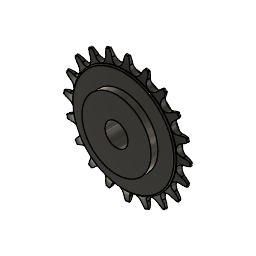
2410994757_Bicycle-sprocket1 (Autodesk Fusion 360 design; units mm, degrees)
part number: 2025-11-01-18-05-41-506
Autodesk Fusion 360 part; units mm, degrees
sketch "Sketch1" plane through (0, 0, 0) normal (0, 1, 0) x (1, 0, 0)
  circle A0 centre (0, 0) radius 37.5
  circle A1 centre (0, 0) radius 33.75
  circle A2 centre (0, 0) radius 41.6667
  line L0 (0, 0) -> (0, -48.246)
  line L1 (0, 0) -> (-7.6961, -48.5915)
  circle A3 centre (-5.8663, -37.0383) radius 3.75
  circle A4 centre (5.8663, -37.0383) radius 3.75
  circle A5 centre (9.5362, -36.2672) radius 11.6717
  circle A6 centre (-9.5362, -36.2672) radius 11.6717
  arc A7 (-1.0259, -41.2344) -> (-0.3536, -41.6652) centre (-0.3472, -40.9152) ccw
  arc A8 (0.3536, -41.6652) -> (1.0259, -41.2344) centre (0.3472, -40.9152) ccw
  dimension "d1" = 75
  dimension "d3" = 67.5
  dimension "d4" = 83.3333
  dimension "d5" = 9
  dimension "d6" = 1.5
  constraint coincident A0.centre A1.centre
  constraint concentric A0 A1
  constraint concentric A1 A2
  constraint vertical L0
  constraint coincident A0 A3.centre
  constraint coincident L1 A3.centre
  constraint tangent A1 A3
  constraint symmetric L0 A3 A4
  constraint coincident A4 A5.centre
  constraint coincident A0 A5.centre
  constraint tangent A3 A5
  constraint symmetric L0 A5 A6
  constraint tangent A5 A7
  constraint tangent A2 A7
  constraint symmetric L0 A7 A8
  constraint coincident A5 A7.start
  constraint coincident A6 A8.end
  constraint coincident A2 A7.end
  constraint coincident A2 A8.start
  measures "d1" diameter of A0
  measures "d3" diameter of A1
  measures "d4" diameter of A2
  measures "d5" angle of L0 L1
  measures "d6" diameter of A7
extrude "Extrude1" add sketch "Sketch1" along normal mid plane 6 contours A1 A3 A5 | A1 A4 A6 | A0 A1 L0 A5 | A0 A2 L0 A6 A8 | A0 A1 L0 A6 | A0 A2 L0 A5 A7 makes body 1
extrude "Extrude2" add sketch "Sketch1" along normal mid plane 6 separate body contours A1 L1 A6 | A1 L0 L1 A5 A6 | A1 A5 A6 | A1 L1 A5 A6 | L0 L1 A6 | A1 L0 A6 | A1 L0 A5 makes body 2
sketch "Sketch2" plane through (0, 0, 0) normal (1, 0, 0) x (0, 1, 0)
  line L0 (0, 0) -> (0, 50)
  line L1 (3, 0) -> (3, 60)
  line L2 (-3, 0) -> (-3, 60)
  arc A0 (-2.0965, 33.3228) -> (-0.6531, 41.0213) centre (-23.3532, 41.2928) ccw
  arc A1 (0.6531, 41.0213) -> (2.0965, 33.3228) centre (23.3532, 41.2928) ccw
  circle A2 centre (0, 0) radius 33.75
  line L3 (-9, 52) -> (-8, 52)
  line L4 (-8, 52) -> (27, 52)
  arc A3 (-3, 41.5585) -> (3, 41.5585) centre (0, 0) ccw
  arc A4 (0, 41.6667) -> (-0.6545, 41.6615) centre (0, 0) ccw
  line L5 (0, 0) -> (-0.5301, 33.7458)
  line L6 (-0.6543, 41.6494) -> (-0.7647, 48.6769)
  arc A5 (0.6531, 41.0213) -> (-0.6531, 41.0213) centre (0, 41.0135) ccw
  line L7 (-50, 0) -> (55, 0)
  dimension "d11" = 0.9
  dimension "d13" = 83.3333
  dimension "d14" = 67.5
  constraint coincident L0.start A2.centre
  constraint vertical L0
  constraint symmetric L0 L1.start L2.start
  constraint symmetric L0 L1.end L2.end
  constraint tangent A0 L5
  constraint coincident L6.start L5
  constraint symmetric L0 A0.start A1.end
  constraint symmetric L0 A0 A1
  constraint horizontal L3
  constraint parallel L3 L4
  constraint coincident L0 A5.centre
  constraint tangent A0 A5
  constraint tangent A3 A5
  constraint coincident A4.end L5
  constraint coincident L2 A3.start
  constraint coincident L1 A3.end
  constraint coincident L0 A4.start
  constraint concentric A3 A4
  constraint collinear L5 L6
  constraint coincident A2 L5.end
  constraint horizontal L7
  measures "d11" angle of L0 L5
  measures "d13" diameter of A3
  measures "d14" diameter of A2
revolve "Revolve1" cut sketch "Sketch2" angle 360 about axis through (0, -50, 0) along (0, 1, 0) contours L1 L2 A0 A1 A2 L4 A5 | L2 A2 A3 L7 | L1 A2 A3 L7 bodies 1 2
fillet "Fillet1" radius 0.75 2 edges at (12.1562, -3, -31.3415) (12.1562, 3, 31.3415) on bodies 2
sketch "Sketch3" plane through (0, 0, 0) normal (0, 1, 0) x (1, 0, 0)
  circle A0 centre (0, 0) radius 7.5
  circle A1 centre (0, 0) radius 22.5
  dimension "d18" = 15
  dimension "d19" = 45
  constraint coincident A0.centre A1.centre
  measures "d18" diameter of A0
  measures "d19" diameter of A1
extrude "Extrude3" add sketch "Sketch3" along normal mid plane 15 separate body makes body 3
extrude "Extrude4" cut sketch "Sketch3" along normal mid plane 40 contours A0 bodies 2
pattern_circular "C-Pattern1" count 20 over 360 about axis through (0, -3, 0) along (0, 1, 0) of bodies 1 makes body 4 at (6.4398, 0.6471, 33.1299) makes body 5 at (17.3825, -0.6471, 28.9294) makes body 6 at (28.9294, 0.6471, 17.3825) makes body 7 at (31.067, -0.6471, 13.1872) makes body 8 at (33.6216, -0.6471, 2.9415) makes body 9 at (33.1299, 0.6471, -6.4398) makes body 10 at (29.5184, 0.6471, -16.3623) makes body 11 at (22.142, -0.6471, -25.4714) makes body 12 at (13.1872, -0.6471, -31.067) makes body 13 at (2.9415, -0.6471, -33.6216) makes body 14 at (-7.5921, -0.6471, -32.885) makes body 15 at (-16.3623, 0.6471, -29.5184) makes body 16 at (-25.4714, -0.6471, -22.142) makes body 17 at (-31.067, -0.6471, -13.1872) makes body 18 at (-33.6216, -0.6471, -2.9415) makes body 19 at (-32.885, -0.6471, 7.5921) makes body 20 at (-28.9294, -0.6471, 17.3825) makes body 21 at (-22.142, -0.6471, 25.4714) makes body 22 at (-13.1872, -0.6471, 31.067)
combine "Combine1" operation add target body 12 tool bodies 4 8 11 18 14 2 15 1 19 3 5 22 20 13 16 9 17 10 7 21 6
equation "d3 = ( 75 * 0.9 ) * 1 mm"
equation "d4 = ( 75 / 0.9 ) * 1 mm"
equation "d7 = 2 * 1.5 mm"
equation "d9 = 2 * 1.5 mm"
equation "d13 = ( 75 / 0.9 ) * 1 mm"
equation "d14 = ( 75 * 0.9 ) * 1 mm"
